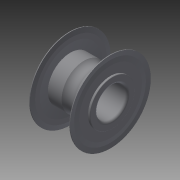
# Autodesk Inventor part: W 639/2-2Z_PART1
Saved by Autodesk Inventor 2014 SP2 (Build 180246200, 246)
## iProperties
Created: 2018-11-24
Part Number: W 639/2-2Z_PART1
Material: Generic
Catalog Web Link: www.cadenas.de
Description: -Deep groove ball bearings
Vendor: SKF
Document SubType Name: Modeling
Designer: psadmin
Manufacturer: SKF
Mass: 0.0131184 g
Surface Area: 1.18292 cm^2
Volume: 0.0131184 cm^3
Density: 1 g/cm^3
Appearance: PSOLRGB-175-175-175
Category: PARTsolutions
Company: SKF
Title: W 639/2-2Z_PART1
Author: Cadenas PARTsolutions
Comments: Deep groove ball bearings
PSOL_IDENT_0: {$CADENAS_DATA\23d-libs\skf\bearings_units_and_housings\ball_bearings\deep_groove_ball_bearings\bb1_
PSOL_IDENT_1: 001_101.prj},199 {VTYP=3D},{NB=W 639/2-2Z_PART1},{LINA=W 639/2-2Z_PART1},{NN=BB1_001_101_PART1},{NOP
PSOL_IDENT_2: RJ=TRUE},{DATE=05.11.2018 07:58:23},{GEOMDATE=08.08.2018 12:16:40},{VERSION=},{LINEID=18460},{WBVAR=
PSOL_IDENT_3: },{WBNUMERIC=}  {NB=W 639/2-2Z_PART1},{LINA=W 639/2-2Z_PART1},{KT=DUMMY},{PRODUCTID=1010476392},{DES
PSOL_IDENT_4: IGNATION=W 639/2-2Z},{DD=2.00},{D=6.000},{B=3.000},{C=0.000},{DD1=3.00},{DD2=0.0},{D1=0.00},{D2=5.40
PSOL_IDENT_5: },{D3=0.00},{D4=0.000},{HH=MIN},{BB=0.000},{FF=0.00},{R0MAX=MIN},{R0=MIN},{R12=0.15},{PITCH=3.90},{D
PSOL_IDENT_6: W=1.200},{DDAMIN=2.900},{DDAMAX=2.900},{DDBMIN=MIN},{DDBMAX=MIN},{DBMIN=MIN},{DAMAX=5.400},{BBAMIN=M
PSOL_IDENT_7: IN},{CAMAX=MIN},{RAMAX=0.150},{LOAD1=0.190},{LOAD2=0.051},{LOAD3=0.002},{SPEED1=180000},{SPEED2=9000
PSOL_IDENT_8: 0},{KR=0.025},{F0=6.000},{Z=6},{II=1},{MASS=0.000},{BEARING=W 639/2-2Z},{RING=},{HELP=0.648},{HELP2=
PSOL_IDENT_9: 0.300},{DD1ALG=1.500},{YALG=1.500},{PITCH1=3.900},{DW1=1.200},{YALG1=2.352},{HALG1=0.648},{SH=1.500}
PSOL_IDENT_10: ,{CU=0.360},{DESIGN=dgbbw2z},{HALG=0.5},{B1=0},{ALGO=1.000}
NT: Deep groove ball bearings
NB: W 639/2-2Z_PART1
NBSYN: $DESIGNATION._PART1
LINA: W 639/2-2Z_PART1
SUPPLIER: SKF
ARTICLENO: W 639/2-2Z_PART1
BOMINFO: W 639/2-2Z_PART1
CREATOR: CADENAS GmbH
Autodesk Inventor part; units mm, degrees
ref_plane "YZ Plane" through (0, 0, 0) normal (1, 0, 0) x (0, 1, 0)
ref_plane "XZ Plane" through (0, 0, 0) normal (0, 1, 0) x (-1, 0, 0)
ref_plane "XY Plane" through (0, 0, 0) normal (0, 0, 1) x (1, 0, 0)
sketch "Sketch_17" plane through (0, 0, 0) normal (0, 0, 1) x (1, 0, 0)
  line L0 (50, 0) -> (-50, 0)
  line L1 (0, 1.47) -> (0, 1.15)
  arc A0 (0, 1.15) -> (0.15, 1) centre (0.15, 1.15) ccw
  line L2 (0.15, 1) -> (2.85, 1)
  arc A1 (2.85, 1) -> (3, 1.15) centre (2.85, 1.15) ccw
  line L3 (3, 1.15) -> (3, 1.47)
  arc A2 (3, 1.47) -> (2.97, 1.5) centre (2.97, 1.47) ccw
  line L4 (2.97, 1.5) -> (1.8969, 1.5)
  arc A3 (1.1031, 1.5) -> (1.8969, 1.5) centre (1.5, 1.95) ccw
  line L5 (1.1031, 1.5) -> (0.03, 1.5)
  arc A4 (0.03, 1.5) -> (0, 1.47) centre (0.03, 1.47) ccw
  constraints: 12 end point, 10 point on circle, 5 centre point
revolve "Revolution1" add sketch "Sketch_17" angle 360 about axis through (50, 0, 0) along (1, 0, 0)
sketch "Sketch_20" plane through (0, 0, 0) normal (0, 0, 1) x (1, 0, 0)
  line L0 (50, 0) -> (-50, 0)
  line L1 (0.135, 2.7) -> (0.1575, 2.3975)
  line L2 (0.1575, 2.3975) -> (0.135, 2.095)
  line L3 (0.135, 2.095) -> (0.135, 1.49)
  line L4 (0.135, 1.49) -> (0.18, 1.49)
  line L5 (0.18, 1.49) -> (0.225, 2.095)
  line L6 (0.225, 2.095) -> (0.225, 2.3975)
  line L7 (0.225, 2.3975) -> (0.18, 2.7)
  line L8 (0.18, 2.7) -> (0.135, 2.7)
  constraints: 18 end point
revolve "Revolution2" add sketch "Sketch_20" angle 360 about axis through (50, 0, 0) along (1, 0, 0)
sketch "Sketch_21" plane through (0, 0, 0) normal (0, 0, 1) x (1, 0, 0)
  line L0 (50, 0) -> (-50, 0)
  line L1 (2.775, 2.3975) -> (2.775, 2.095)
  line L2 (2.775, 2.095) -> (2.82, 1.49)
  line L3 (2.82, 1.49) -> (2.865, 1.49)
  line L4 (2.865, 1.49) -> (2.865, 2.095)
  line L5 (2.865, 2.095) -> (2.8425, 2.3975)
  line L6 (2.8425, 2.3975) -> (2.865, 2.7)
  line L7 (2.865, 2.7) -> (2.82, 2.7)
  line L8 (2.82, 2.7) -> (2.775, 2.3975)
  constraints: 18 end point
revolve "Revolution3" add sketch "Sketch_21" angle 360 about axis through (50, 0, 0) along (1, 0, 0)
body "Solid1"
